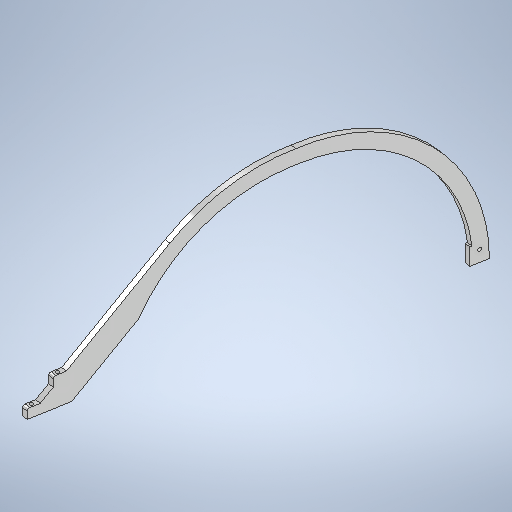
# Autodesk Inventor part: hand2_05
Saved by Autodesk Inventor 2025.1 (Build 291241000, 241)
## iProperties
Created: 2025-02-02
Part Number: hand2_05
Material: アルミニウム 6061-AHC
Document SubType Name: Modeling
Designer: ryogo
Density: 2.7 g/cm^3
Appearance: アルミニウム - ダーク
Author: ryogo
Autodesk Inventor part; units mm, degrees
ref_plane "YZ Plane" through (0, 0, 0) normal (1, 0, 0) x (0, 1, 0)
ref_plane "XZ Plane" through (0, 0, 0) normal (0, 1, 0) x (-1, 0, 0)
ref_plane "XY Plane" through (0, 0, 0) normal (0, 0, 1) x (1, 0, 0)
sketch "スケッチ1" plane through (0, 0, 0) normal (0, 1, 0) x (-1, 0, 0)
  circle A0 centre (0, 0) radius 122.5
  line L0 (0, 0) -> (21.2719, 120.6389)
  line L1 (21.2719, 120.6389) -> (-21.2719, -120.6389)
  line L2 (21.2719, 120.6389) -> (-41.166, -233.4643)
  arc A1 (21.2719, 120.6389) -> (0, 122.5) centre (0, 0) ccw
  arc A2 (-21.2719, -120.6389) -> (0, -122.5) centre (0, 0) ccw
  arc A3 (-41.8975, -115.1123) -> (-21.2719, -120.6389) centre (0, 0) ccw
  circle A4 centre (0, 0) radius 125
  circle A5 centre (0, 0) radius 145
  arc A6 (-42.7525, -117.4616) -> (-105.9051, -66.4011) centre (0, 0) ccw
  line L3 (0, 0) -> (-42.7525, -117.4616) construction
  line L4 (21.706, 123.101) -> (21.706, 123.101)
  line L5 (0, -145) -> (0, -265.735)
  line L6 (0, 0) -> (-41.8975, -115.1123)
  line L7 (-49.5929, -136.2554) -> (-41.8975, -115.1123)
  line L8 (-42.7525, -117.4616) -> (-231.4975, -48.764)
  line L9 (42.7525, 117.4616) -> (0, 0)
  line L10 (0, -145) -> (0, 145)
  line L11 (0, 0) -> (0, 300)
  circle A7 centre (0, 300) radius 20
  line L12 (117.0937, 43.75) -> (18.735, 307)
  line L13 (0, 0) -> (185.4327, 0)
  line L14 (0, 0) -> (-259.4726, 94.4403)
  line L15 (42.7525, 117.4616) -> (-253.7236, 225.3701)
  line L16 (0, 125) -> (22.0409, 125)
  line L17 (21.2719, 120.6389) -> (25.179, 142.7971)
  line L18 (42.7525, 117.4616) -> (65.8461, 180.9106)
  line L19 (15, 170) -> (69.9226, 170)
  line L20 (15.9946, 175) -> (68.0545, 175)
  line L21 (0, 125) -> (-15, 125)
  line L22 (-15, 125) -> (-15, 325)
  line L23 (-15, 325) -> (0, 325)
  line L24 (0, 325) -> (0, 125)
  line L25 (0, 125) -> (15, 125)
  line L26 (15, 125) -> (15, 325)
  line L27 (15, 325) -> (0, 325)
  line L28 (0, 325) -> (0, 125)
  line L29 (15, 200) -> (15, 325)
  line L30 (15, 325) -> (-15, 325)
  line L31 (-15, 325) -> (-15, 150)
  line L32 (15, 170) -> (37.5, 170)
  line L33 (37.5, 170) -> (17.5, 170)
  line L34 (0, 0) -> (0, 300)
  line L35 (0, -125) -> (42.7525, 117.4616)
  line L36 (-42.7525, -117.4616) -> (0, 125)
  line L37 (0, -125) -> (-3.519, -144.9573)
  line L38 (42.7525, 117.4616) -> (49.5929, 136.2554)
  line L39 (0, 125) -> (3.519, 144.9573)
  line L40 (-42.7525, -117.4616) -> (-46.2715, -137.4189)
  line L41 (42.7525, 117.4616) -> (46.2715, 137.4189)
  line L42 (-3.519, -144.9573) -> (46.2715, 137.4189)
  line L43 (46.2715, 137.4189) -> (37.2054, 139.0175)
  line L44 (-12.5852, -143.3587) -> (-3.519, -144.9573)
  line L45 (-46.2715, -137.4189) -> (3.519, 144.9573)
  line L46 (3.519, 144.9573) -> (12.5852, 143.3587)
  line L47 (-37.2054, -139.0175) -> (-46.2715, -137.4189)
  line L48 (-27.6373, -142.3418) -> (-22.7132, -143.21)
  line L49 (-27.6373, -142.3418) -> (-22.7132, -143.21)
  line L50 (-22.7132, -143.21) -> (27.641, 142.363)
  line L51 (27.641, 142.363) -> (22.717, 143.2312)
  line L52 (22.717, 143.2312) -> (-27.6373, -142.3418)
  line L53 (12.5852, 143.3587) -> (-37.2054, -139.0175)
  line L54 (-12.5852, -143.3587) -> (37.2054, 139.0175)
  line L55 (-42.1294, -138.1492) -> (7.6611, 144.2269)
  line L56 (-7.6611, -144.2269) -> (42.1294, 138.1492)
  line L57 (12.5852, 143.3587) -> (7.6611, 144.2269)
  line L58 (7.6611, 144.2269) -> (29.236, 266.5842)
  line L59 (29.236, 266.5842) -> (34.1601, 265.7159)
  line L60 (34.1601, 265.7159) -> (12.5852, 143.3587)
  line L61 (22.717, 143.2312) -> (25.179, 142.7971)
  line L62 (25.179, 142.7971) -> (42.462, 240.8141)
  line L63 (42.462, 240.8141) -> (40, 241.2482)
  line L64 (40, 241.2482) -> (22.717, 143.2312)
  line L65 (42.1294, 138.1492) -> (37.2054, 139.0175)
  line L66 (37.2054, 139.0175) -> (49.9319, 211.1932)
  line L67 (49.9319, 211.1932) -> (54.8559, 210.3249)
  line L68 (54.8559, 210.3249) -> (42.1294, 138.1492)
  line L69 (25.179, 142.7971) -> (27.641, 142.363)
  line L70 (27.641, 142.363) -> (44.508, 238.0204)
  line L71 (44.508, 238.0204) -> (42.046, 238.4546)
  line L72 (42.046, 238.4546) -> (25.179, 142.7971)
  line L73 (15.9946, 175) -> (15, 175)
  line L74 (15, 175) -> (0, 175)
  line L75 (0, 175) -> (0, 170)
  line L76 (0, 170) -> (15, 170)
  line L77 (15, 170) -> (15, 175)
  line L78 (20, 175) -> (40, 175)
  line L79 (40, 175) -> (40, 245)
  line L80 (40, 245) -> (20, 245)
  line L81 (20, 245) -> (20, 175)
  line L82 (30, 175) -> (30, 118.7697)
  line L83 (0, 175) -> (58.7137, 175)
  line L84 (58.7137, 175) -> (58.7137, 200)
  line L85 (58.7137, 200) -> (0, 200)
  line L86 (0, 200) -> (0, 175)
  line L87 (0, 200) -> (50, 200)
  line L88 (50, 200) -> (50, 170)
  line L89 (50, 170) -> (0, 170)
  line L90 (0, 170) -> (0, 200)
  line L91 (50, 170) -> (0, 170)
  line L92 (0, 170) -> (0, 165)
  line L93 (0, 200) -> (-15, 200)
  line L94 (-15, 200) -> (-15, 180)
  line L95 (-15, 180) -> (0, 180)
  line L96 (0, 180) -> (0, 200)
  line L97 (0, 180) -> (-15, 180)
  line L98 (-15, 180) -> (-15, 175)
  line L99 (-15, 175) -> (0, 175)
  line L100 (0, 175) -> (0, 180)
  line L101 (0, 145) -> (-15, 145)
  line L102 (-15, 145) -> (-20.5, 145)
  line L103 (-20.5, 145) -> (-20.5, 200)
  line L104 (-20.5, 200) -> (-15, 200)
  line L105 (-15, 200) -> (-15, 145)
  line L106 (-20.5, 150) -> (-25, 150)
  line L107 (-25, 150) -> (-25, 180)
  line L108 (-25, 180) -> (-20.5, 180)
  line L109 (-20.5, 180) -> (-20.5, 150)
  line L110 (50, 175) -> (-15, 175)
  line L111 (-15, 175) -> (-15, 170)
  line L112 (50, 170) -> (50, 175)
  line L113 (-20.5, 165) -> (-25, 165)
  line L114 (-25, 165) -> (-25, 195)
  line L115 (-25, 195) -> (-20.5, 195)
  line L116 (-20.5, 195) -> (-20.5, 165)
  line L117 (15, 250) -> (-15, 250)
  line L118 (-15, 145) -> (15, 145)
  line L119 (31.698, 266.1501) -> (-39.6674, -138.5834)
  line L120 (52.3939, 210.7591) -> (-10.1232, -143.7928)
  line L121 (49.3441, 179.0659) -> (14.8758, 185.1436)
  line L122 (-15, 138.4818) -> (-15, 121.5782)
  line L123 (-7.6611, -144.2269) -> (-42.1294, -138.1492)
  line L124 (-39.6243, -123.9424) -> (-5.1561, -130.02)
  line L125 (-42.2291, -138.7145) -> (-7.7608, -144.7922)
  line L126 (-41.3608, -133.7904) -> (-6.8926, -139.8681)
  line L127 (-6.0243, -134.9441) -> (-40.4926, -128.8664)
  line L128 (18.3488, 204.8397) -> (52.8171, 198.762)
  line L129 (50.2124, 183.9899) -> (45.0029, 154.4457)
  line L130 (10.5346, 160.5234) -> (15.7441, 190.0676)
  line L131 (19.217, 209.7638) -> (53.6853, 203.6861)
  line L132 (15, 250) -> (53.6853, 203.6861)
  line L133 (53.6853, 203.6861) -> (53.6853, 170)
  line L134 (53.6853, 170) -> (-15, 170)
  line L135 (-15, 172.5) -> (53.6853, 172.5)
  line L136 (15, 170) -> (15, 150)
  line L137 (15, 150) -> (-15, 150)
  line L138 (-15, 170) -> (15, 170)
  line L139 (15, 150) -> (-15, 150)
  line L140 (-15, 150) -> (-15, 325)
  line L141 (-15, 325) -> (15, 325)
  line L142 (15, 325) -> (15, 150)
  circle A8 centre (0, 300) radius 6
  circle A9 centre (0, 300) radius 11
  line L143 (47.7456, 170) -> (15, 150)
  point P0 (-25.1752, -142.7759)
  point P1 (42.3116, 114.9608)
  point P2 (0, 133.0222)
  point P3 (-38.8988, -134.2246)
  point P4 (-38.0306, -129.3005)
  point P5 (-23.2585, -131.9052)
  point P6 (-24.1267, -136.8293)
  point P7 (-9.3546, -139.434)
  point P8 (-8.4863, -134.51)
  point P9 (17.3379, 184.7094)
  point P10 (32.11, 182.1047)
  point P11 (46.8821, 179.5)
  point P12 (50.3551, 199.1962)
  point P13 (35.5829, 201.8009)
  point P14 (20.8108, 204.4056)
  point P15 (0, 240)
  point P16 (0, 190)
  point P17 (0, 289)
  point P18 (0, 311)
  point P19 (37.5, 172.5)
  point P20 (22.5, 172.5)
  point P21 (42.6684, 170)
  point P22 (47.7456, 170)
  point P23 (48.7613, 204.5543)
  point P24 (-10.0801, -129.1518)
  dimension "d0" = 245
  dimension "d7" = 290
  dimension "d19" = 40
  dimension "d1" = 0
  dimension "d4" = 42.5438
  dimension "d5" = 21.3532
  dimension "d6" = 250
  dimension "d10" = 0
  dimension "d12" = 0
  dimension "d13" = 10
  dimension "d15" = 0
  dimension "d16" = 9.8877
  dimension "d18" = 10
  dimension "d21" = 145
  dimension "d23" = 175
  dimension "d26" = 7.5384
  dimension "d30" = 180
  dimension "d34" = 180
  dimension "d35" = 45
  dimension "d37" = 5
  dimension "d38" = 15
  dimension "d39" = 200
  dimension "d40" = 15
  dimension "d41" = 200
  dimension "d47" = 300
  dimension "d52" = 5
  dimension "d53" = 0
  dimension "d54" = 10
  dimension "d55" = 10
  dimension "d56" = 5
  dimension "d57" = 5
  dimension "d60" = 5
  dimension "d61" = 20
  dimension "d62" = 70
  dimension "d63" = 5
  dimension "d65" = 25
  dimension "d66" = 50
  dimension "d68" = 20
  dimension "d69" = 5
  dimension "d74" = 20
  dimension "d75" = 5.5
  dimension "d76" = 55
  dimension "d77" = 4.5
  dimension "d78" = 30
  dimension "d79" = 5
  dimension "d82" = 15
  dimension "d83" = 50
  dimension "d87" = 16.9036
  dimension "d88" = 10.0392
  dimension "d89" = 10.5222
  dimension "d92" = 15
  dimension "d93" = 5
  dimension "d94" = 5
  dimension "d96" = 4.5
  dimension "d97" = 5
  dimension "d98" = 30
  dimension "d99" = 10
  dimension "d101" = 20
  dimension "d102" = 10
  dimension "d103" = 20
  dimension "d104" = 12
  dimension "d105" = 22
  dimension "d106" = 7.5
  dimension "d107" = 15
  dimension "d108" = 30
  constraints: 287 end point, 87 point on line, 44 parallel, 39 perpendicular, 19 horizontal, 16 point on circle, 14 midpoint, 9 coincident, 9 collinear, 7 centre point, 3 vertical, 2 tangent, 1 symmetric about line, 43 other
  measures "d1" horizontal distance of point (0, 0) A2.end
  measures "d4" distance of L6.end A2.end
  measures "d5" distance of A1.end L0.end
  measures "d6" diameter of A4
  measures "d10" horizontal distance of A4.centre L16.start
  measures "d12" distance from line of L5 point (0, 0)
  measures "d15" horizontal distance of A2.end L35.start
  measures "d16" vertical distance of L6.end L35.start
  measures "d18" angle of L9 L1
  measures "d21" distance of L5.start A2.centre
  measures "d23" distance of L11.end L16.start
  measures "d26" distance from line of L15 L16.start
  measures "d30" angle of L4 L17
  measures "d34" angle of L9 L18
  measures "d35" distance from line of L19 L16.start
  measures "d37" distance between parallel lines of L19 L20
  measures "d38" distance of L22.end L23.end
  measures "d39" distance of L21.end L22.end
  measures "d40" distance of L27.end L26.end
  measures "d41" distance from line of L16.start L27
  measures "d47" distance of L3.start L11.end
  measures "d52" distance of L48.start L48.end
  measures "d53" distance from line of L2 point (-25.175, -142.776)
  measures "d54" distance between parallel lines of L52 L53
  measures "d55" distance between parallel lines of L54 L50
  measures "d56" distance of L46.end L55.end
  measures "d57" distance of L43.end L56.end
  measures "d60" distance between parallel lines of L76 L74
  measures "d61" distance of L80.end L79.end
  measures "d62" distance of L79.end L78.end
  measures "d63" distance between parallel lines of L26 L81
  measures "d65" distance of L84.end L83.end
  measures "d66" distance of L88.end L89.end
  measures "d68" distance between parallel lines of L95 L93
  measures "d69" distance between parallel lines of L99 L97
  measures "d74" distance of L16.start L101.start
  measures "d75" distance of L103.end L104.end
  measures "d76" distance of L102.end L103.end
  measures "d77" distance of L107.end L108.end
  measures "d78" distance of L106.end L107.end
  measures "d79" distance between parallel lines of L102 L106
  measures "d82" distance between parallel lines of L106 L113
  measures "d83" distance between parallel lines of L93 L117
  measures "d87" distance of L122.start L122.end
  measures "d88" vertical distance of point (42.312, 114.961) L25.end
  measures "d89" distance of A1.end point (0, 133.022)
  measures "d92" distance of L125.start L124.start
  measures "d93" distance of L125.start L126.start
  measures "d94" distance of L127.end L124.start
  measures "d96" distance from line of L20 point (46.882, 179.5)
  measures "d97" distance of L121.end L130.end
  measures "d98" distance of L129.start L129.end
  measures "d99" distance from line of L117 point (0, 240)
  measures "d101" distance of L128.start L121.end
  measures "d102" diameter of L131 L128
  measures "d103" distance of L19.start L136.end
  measures "d104" diameter of A8
  measures "d105" diameter of A9
  measures "d106" distance from line of point (22.5, 172.5) L142
  measures "d107" distance of point (22.5, 172.5) point (37.5, 172.5)
  measures "d108" distance between parallel lines of L113 L115
extrude "押し出し1" add sketch "スケッチ1" along normal blind 5 contours L56 L127 L120 L124 | L44 L120 L126 L56 | L120 L127 L54 L124 | L56 L126 L120 L127 | L44 L54 L126 L120 | L19 L120 L135 L68 | L120 L126 L54 L127 | L19 L66 L135 L120 | L135 L120 L20 L68 | L135 L66 L20 L120 | L20 L120 L121 L68 | L68 L85 L120 L131 | L68 L128 L120 L85 | L88 L120 L128 L68 | L68 L121 L120 L88 | L20 L66 L121 L120 | L120 L85 L66 L131 | L120 L128 L88 L85 | L120 L121 L66 L128 L88 | L88 L128 L120 | L88 L128 L66 L85
sketch "スケッチ3" plane through (-42.6684, 0, 170) normal (0.9848078, 0, 0.1736482) x (0.1736482, 0, -0.9848078)
  line L0 (319.8266, 0) -> (29.8266, 0) projected
  circle A0 centre (174.8266, 0) radius 125
  circle A1 centre (167.3266, 0) radius 132.5
  circle A2 centre (174.8266, 0) radius 132.5
  circle A3 centre (174.8266, 0) radius 145
  circle A4 centre (167.3266, 0) radius 145
  line L1 (174.8266, 145) -> (167.3266, 145)
  line L2 (174.8266, 132.5) -> (167.3266, 132.5)
  line L3 (-35.0874, 0) -> (-35.0874, 5) projected
  line L4 (319.8266, 0) -> (-35.0874, 0)
  point P0 (319.8266, 0)
  point P1 (171.0766, 144.9515)
  point P2 (22.3266, 0)
  point P3 (29.8266, 0)
  point P4 (34.8266, 0)
  point P5 (307.3266, 0)
  dimension "d113" = 265
  dimension "d114" = 265
  dimension "d116" = 290
  dimension "d112" = 250
  dimension "d115" = 290
  constraints: 6 end point, 4 coincident, 4 horizontal, 2 centre point, 2 point on circle, 1 point on line, 1 tangent, 10 other
  measures "d112" diameter of A0
  measures "d115" diameter of A3
extrude "押し出し2" add sketch "スケッチ3" against normal blind 5 contours L0 A4 A3 | L0 A2 L2 A1 A3 A4 | A3 L4 A4 picked at (317.0227, 5.4116) picked at (25.1305, 5.4116)
sketch "スケッチ4" plane through (-18.5365, 0, 4.3472) normal (-0.9848078, 0, -0.1736482) x (-0.1243654, -0.6979033, 0.7053115)
  line L0 (120.4694, 117.3931) -> (144.9673, 141.2654) projected
  line L1 (94.8954, 92.4722) -> (144.9673, 141.2654)
  line L2 (144.9673, 141.2654) -> (134.4987, 152.0083)
  line L3 (134.4987, 152.0083) -> (84.4269, 103.2151)
  line L4 (84.4269, 103.2151) -> (94.8954, 92.4722)
  line L5 (84.4269, 103.2151) -> (83.7872, 102.5917)
  arc A0 (103.8478, 101.196) -> (-103.8478, 101.196) centre (0, 0) ccw projected
  line L6 (116.3485, 120.3587) -> (116.9799, 120.974) projected
  line L7 (144.9673, 141.2654) -> (131.0092, 155.5892)
  line L8 (131.0092, 155.5892) -> (106.5113, 131.7169)
  line L9 (106.5113, 131.7169) -> (120.4694, 117.3931)
  line L10 (120.4694, 117.3931) -> (144.9673, 141.2654)
  line L11 (120.4694, 117.3931) -> (116.9799, 120.974) projected
  line L12 (131.0092, 155.5892) -> (106.5113, 131.7169)
  line L13 (106.5113, 131.7169) -> (106.5113, 131.7169)
  line L14 (106.5113, 131.7169) -> (131.0092, 155.5892)
  line L15 (131.0092, 155.5892) -> (131.0092, 155.5892)
  line L16 (131.0092, 155.5892) -> (-11.2051, 144.5664)
  line L17 (106.5113, 131.7169) -> (66.8962, 128.6464)
  line L18 (127.0625, 123.8178) -> (113.1044, 138.1416)
  line L19 (141.3863, 137.7759) -> (127.4283, 152.0997)
  line L20 (137.8054, 134.2863) -> (118.027, 154.583)
  line L21 (118.027, 154.583) -> (125.1889, 161.562)
  line L22 (125.1889, 161.562) -> (144.9673, 141.2654)
  line L23 (144.9673, 141.2654) -> (137.8054, 134.2863)
  line L24 (116.9799, 120.974) -> (141.4778, 144.8463) projected
  line L25 (119.992, 123.9092) -> (92.0626, 152.5705)
  line L26 (92.0626, 152.5705) -> (99.2245, 159.5496)
  line L27 (99.2245, 159.5496) -> (127.1539, 130.8883)
  line L28 (127.1539, 130.8883) -> (119.992, 123.9092)
  line L29 (106.5113, 131.7169) -> (39.3775, 126.5135)
  arc A1 (94.8954, 92.4722) -> (-92.4722, 94.8954) centre (0, 0) ccw projected
  point P0 (-5.3714, -5.2343)
  point P1 (141.3863, 137.7759)
  point P2 (131.0092, 155.5892)
  point P3 (106.5113, 131.7169)
  point P4 (131.0092, 155.5892)
  point P5 (105.0448, 153.5768)
  point P6 (66.8962, 128.6464)
  point P7 (110.0009, 128.136)
  point P8 (92.8221, 111.3959)
  point P9 (120.4694, 117.3931)
  dimension "d119" = 15
  dimension "d121" = 20
  dimension "d122" = 0
  dimension "d123" = 0
  dimension "d124" = 10
  dimension "d125" = 0
  dimension "d126" = 10
  dimension "d127" = 5
  dimension "d128" = 0
  constraints: 52 end point, 11 parallel, 9 perpendicular, 8 point on line, 3 point on circle, 1 collinear, 1 midpoint, 1 tangent, 2 other
  measures "d119" distance of L2.end L1.end
  measures "d121" distance of L1.end L7.end
  measures "d122" distance between parallel lines of L9 L11
  measures "d123" distance of L8.end L13.end
  measures "d124" distance from line of L20 point (131.009, 155.589)
  measures "d125" distance between parallel lines of L15 L22
  measures "d126" distance of L25.end L26.end
  measures "d127" distance between parallel lines of L27 L18
  measures "d128" distance between parallel lines of L29 L17
extrude "押し出し3" add sketch "スケッチ4" against normal blind 5 contours A0 L16 L25 L8 L17 | L8 L25 L16 L27 | L20 L16 L8 | L8 L27 L16 L20 | L26 L27 L16 | L21 L22 L16
extrude "押し出し4" cut sketch "スケッチ4" against normal blind 5 contours L1 L4 L3 A0 | A1 L5 L4 | L3 L5 A1 L29 A0
extrude "押し出し5" cut sketch "スケッチ4" against normal blind 5 contours L9 L24 L18 L0 | L1 A0 L3 L9 | L18 L24 L20 L0 | L20 L24 L19 L0 | L19 L24 L2 L0
sketch "スケッチ6" plane through (-12.3101, 0, -2.1706) normal (0.9848078, 0, 0.1736482) x (0.1243654, -0.6979033, -0.7053115)
  arc A0 (103.8478, 101.196) -> (-103.8478, 101.196) centre (0, 0) ccw projected
  line L0 (103.8478, 101.196) -> (92.3459, 89.9877) projected
  line L1 (103.8478, 101.196) -> (94.2854, 91.8777)
  line L2 (94.2854, 91.8777) -> (83.8168, 102.6206)
  line L3 (83.8168, 102.6206) -> (93.3793, 111.9389)
  line L4 (93.3793, 111.9389) -> (103.8478, 101.196)
  line L5 (-139.7989, -108.3035) -> (-132.861, -41.3267) projected
  arc A1 (-97.8436, 89.6612) -> (-132.861, -41.3267) centre (-5.3714, -5.2343) ccw projected
  line L6 (-97.8436, 89.6612) -> (-92.4722, 94.8954) projected
  arc A2 (91.3383, 95.9873) -> (-92.4722, 94.8954) centre (0, 0) ccw projected
  line L7 (88.8564, 93.5687) -> (91.3383, 95.9873) projected
  line L8 (92.3459, 89.9877) -> (88.8564, 93.5687) projected
  line L9 (92.3459, 89.9877) -> (103.8478, 101.196) projected
  arc A3 (103.8478, 101.196) -> (-103.8478, 101.196) centre (0, 0) ccw projected
  arc A4 (-103.8478, 101.196) -> (-149.5997, 9.7059) centre (-5.3714, -5.2343) ccw projected
  line L10 (-149.5997, 9.7059) -> (-160.2719, -93.3203) projected
  line L11 (-160.2719, -93.3203) -> (-167.4338, -100.2993) projected
  line L12 (-167.4338, -100.2993) -> (-161.6135, -106.2721) projected
  line L13 (-161.6135, -106.2721) -> (-162.9551, -119.224) projected
  line L14 (-162.9551, -119.224) -> (-170.1171, -126.203) projected
  line L15 (-170.1171, -126.203) -> (-164.2968, -132.1758) projected
  line L16 (-164.2968, -132.1758) -> (-139.7989, -108.3035) projected
  point P0 (0, 0)
  point P1 (92.8221, 111.3959)
  dimension "d135" = 15
  constraints: 8 end point, 2 parallel, 1 perpendicular, 1 point on circle, 1 point on line
  measures "d135" distance of L1.end L2.end
extrude "押し出し6" add sketch "スケッチ6" against normal blind 5 contours L0 L2 L7 A2 L3 A0 | A2 L7 L2
sketch "スケッチ7" plane through (10.5504, 5, -131.8188) normal (0.9848078, 0, 0.1736482) x (0.1736482, 0, -0.9848078)
  line L0 (0, 0) -> (-2.7081, 0) projected
  line L1 (0, 0) -> (-2.7081, 0)
  line L2 (-2.7081, 0) -> (-2.7081, -5)
  line L3 (-2.7081, -5) -> (0, -5)
  line L4 (0, -5) -> (0, 0)
  point P0 (-131.6482, -5)
  constraints: 8 end point, 2 parallel, 1 horizontal, 1 perpendicular
extrude "押し出し7" cut sketch "スケッチ7" against normal blind 5
sketch "スケッチ8" plane through (10.5504, 0, -131.8188) normal (0.9848078, 0, 0.1736482) x (0.1736482, 0, -0.9848078)
  line L0 (0, 15) -> (0, 0) projected
  line L1 (0, 0) -> (13.3518, 0) projected
  arc A0 (13.3518, 0) -> (-135.3982, 144.9515) centre (-131.6482, 0) ccw projected
  arc A1 (-135.3982, 144.9515) -> (-232.0166, 111.3574) centre (-139.1482, 0) ccw projected
  line L2 (-232.0166, 111.3574) -> (-311.5622, 45.019) projected
  line L3 (-311.5622, 45.019) -> (-321.5622, 45.019) projected
  line L4 (-321.5622, 45.019) -> (-321.5622, 36.6793) projected
  line L5 (-321.5622, 36.6793) -> (-331.5622, 28.3397) projected
  line L6 (-331.5622, 28.3397) -> (-341.5622, 28.3397) projected
  line L7 (-341.5622, 28.3397) -> (-341.5622, 20) projected
  line L8 (-341.5622, 20) -> (-307.3565, 20) projected
  line L9 (-307.3565, 20) -> (-255.6442, 63.1263) projected
  arc A2 (-139.1482, 132.5) -> (-255.6442, 63.1263) centre (-139.1482, 0) ccw projected
  line L10 (-139.1482, 132.5) -> (-131.6482, 132.5) projected
  arc A3 (0, 15) -> (-131.6482, 132.5) centre (-131.6482, 0) ccw projected
  line L11 (13.3518, 0) -> (13.3518, 15)
  line L12 (13.3518, 15) -> (-1.6482, 15)
  line L13 (-1.6482, 15) -> (-1.6482, 0)
  line L14 (-1.6482, 0) -> (13.3518, 0)
  point P0 (-131.6482, 0)
  point P1 (0, 15)
  dimension "d140" = 15
  dimension "d141" = 15
  constraints: 8 end point, 3 parallel, 1 perpendicular, 1 tangent
  measures "d140" distance of L12.end L11.end
  measures "d141" distance between parallel lines of L1 L12
extrude "押し出し8" add sketch "スケッチ8" against normal blind 5 contours L0 L14 L13 L12
sketch "スケッチ9" plane through (-50.2124, 45.019, 183.9899) normal (0, 1, 0) x (0.9848078, 0, 0.1736482)
  line L0 (0, 10) -> (5, 10) projected
  line L1 (2.5, 10) -> (2.5, -20)
  line L2 (0, -20) -> (5, -20) projected
  line L3 (0, 0) -> (5, 0) projected
  point P0 (17.5, 189.914)
  point P1 (2.5, 5)
  point P2 (2.5, -15)
  dimension "d144" = 5
  dimension "d145" = 5
  constraints: 2 end point, 2 midpoint, 2 point on line
  measures "d144" distance from line of L2 point (2.5, -15)
  measures "d145" distance from line of L3 point (2.5, 5)
hole "穴1" at (-46.8821, 45.019, 179.5) at (-50.3551, 45.019, 199.1962) direction (0, -1, 0) diameter 3.1 end through all
fillet "フィレット1" radius 2 2 edges at (-47.7503, 45.019, 184.424) (-51.2233, 28.3397, 204.1202)
sketch "スケッチ10" plane through (10.2642, 0, -130.1956) normal (0.9848078, 0, 0.1736482) x (0.1736482, 0, -0.9848078)
  line L0 (0, 0) -> (0, 15) projected
  line L1 (0, 10) -> (14.6548, 10)
  arc A0 (15, 0) -> (-133.75, 144.9515) centre (-130, 0) ccw projected
  line L2 (0, 0) -> (15, 0) projected
  point P0 (-130, 0)
  point P1 (7.5, 10)
  dimension "d154" = 10
  dimension "d155" = 7.5
  constraints: 2 end point, 2 point on line, 1 horizontal, 1 point on circle
  measures "d154" distance between parallel lines of L2 L1
  measures "d155" distance from line of L0 point (7.5, 10)
hole "穴2" at (11.5665, 10, -137.5817) direction (-0.9848078, 0, -0.1736482) diameter 3.1 end through all
equation "\"d18\" = d13"
